Autodesk Fusion 360 part; units mm, degrees
(part 2 of 3)
  spline S15 degree 5 poles (-10.6114, -19.2717) (-10.6024, -19.2665) (-10.5842, -19.256) (-10.557, -19.2403) (-10.5209, -19.2193) (-10.476, -19.1928) (-10.4312, -19.1661) (-10.3866, -19.1393) (-10.3422, -19.1123) (-10.298, -19.0851) (-10.254, -19.0578) (-10.2102, -19.0302) (-10.1666, -19.0026) (-10.1231, -18.9747) (-10.0799, -18.9466) (-10.0369, -18.9184) (-9.9941, -18.8901) (-9.9515, -18.8615) (-9.9091, -18.8328) (-9.8669, -18.8038) (-9.8249, -18.7748) (-9.7832, -18.7455) (-9.7416, -18.7161) (-9.7003, -18.6865) (-9.6592, -18.6567) (-9.6183, -18.6267) (-9.5776, -18.5966) (-9.5372, -18.5662) (-9.497, -18.5357) (-9.457, -18.5051) (-9.4173, -18.4742) (-9.3778, -18.4432) (-9.3385, -18.412) (-9.2995, -18.3806) (-9.2607, -18.349) (-9.2222, -18.3172) (-9.1839, -18.2853) (-9.1459, -18.2531) (-9.1082, -18.2208) (-9.0707, -18.1883) (-9.0335, -18.1556) (-8.9965, -18.1227) (-8.9598, -18.0896) (-8.9234, -18.0564) (-8.8873, -18.0229) (-8.8515, -17.9892) (-8.816, -17.9554) (-8.7808, -17.9213) (-8.7458, -17.8871) (-8.7112, -17.8526) (-8.6769, -17.8179) (-8.643, -17.7831) (-8.6093, -17.748) (-8.576, -17.7127) (-8.5431, -17.6772) (-8.5105, -17.6415) (-8.4782, -17.6055) (-8.4464, -17.5693) (-8.415, -17.5329) (-8.384, -17.4962) (-8.3534, -17.4593) (-8.3232, -17.4221) (-8.2934, -17.3847) (-8.264, -17.3471) (-8.2352, -17.3092) (-8.2069, -17.2709) (-8.1792, -17.2323) (-8.1523, -17.1934) (-8.1261, -17.154) (-8.1007, -17.1142) (-8.0762, -17.074) (-8.0573, -17.0414) (-8.0434, -17.0168) (-8.0344, -17.0003) (-8.0299, -16.992) knots -1 -1 -1 -1 -1 -1 -0.98571429 -0.97142857 -0.95714286 -0.94285714 -0.92857143 -0.91428571 -0.9 -0.88571429 -0.87142857 -0.85714286 -0.84285714 -0.82857143 -0.81428571 -0.8 -0.78571429 -0.77142857 -0.75714286 -0.74285714 -0.72857143 -0.71428571 -0.7 -0.68571429 -0.67142857 -0.65714286 -0.64285714 -0.62857143 -0.61428571 -0.6 -0.58571429 -0.57142857 -0.55714286 -0.54285714 -0.52857143 -0.51428571 -0.5 -0.48571429 -0.47142857 -0.45714286 -0.44285714 -0.42857143 -0.41428571 -0.4 -0.38571429 -0.37142857 -0.35714286 -0.34285714 -0.32857143 -0.31428571 -0.3 -0.28571429 -0.27142857 -0.25714286 -0.24285714 -0.22857143 -0.21428571 -0.2 -0.18571429 -0.17142857 -0.15714286 -0.14285714 -0.12857143 -0.11428571 -0.1 -0.08571429 -0.07142857 -0.05714286 -0.04285714 -0.02857143 -0.01428571 0 0 0 0 0 0
  line L31 (-8.0299, -16.992) -> (-7.6878, -16.268)
  arc A23 (-7.0347, -16.0238) -> (-7.6878, -16.268) centre (-7.2357, -16.4816) ccw
  arc A24 (-7.0347, -16.0238) -> (-5.868, -16.4869) centre (0, 0) ccw
  arc A25 (-5.5602, -17.1124) -> (-5.868, -16.4869) centre (-6.0357, -16.9579) ccw
  line L32 (-5.5602, -17.1124) -> (-5.8076, -17.874)
  spline S16 degree 5 poles (-5.8076, -17.874) (-5.81, -17.8831) (-5.8148, -17.9013) (-5.8216, -17.9287) (-5.8301, -17.9654) (-5.8399, -18.0115) (-5.8487, -18.0579) (-5.8566, -18.1045) (-5.8637, -18.1513) (-5.8701, -18.1983) (-5.8757, -18.2456) (-5.8807, -18.293) (-5.8852, -18.3405) (-5.8891, -18.3882) (-5.8926, -18.4359) (-5.8957, -18.4838) (-5.8982, -18.5317) (-5.9003, -18.5798) (-5.902, -18.628) (-5.9032, -18.6762) (-5.904, -18.7246) (-5.9043, -18.773) (-5.9043, -18.8216) (-5.9039, -18.8702) (-5.903, -18.9188) (-5.9019, -18.9676) (-5.9003, -19.0164) (-5.8984, -19.0653) (-5.8961, -19.1142) (-5.8935, -19.1632) (-5.8905, -19.2123) (-5.8871, -19.2614) (-5.8835, -19.3106) (-5.8794, -19.3598) (-5.8751, -19.4091) (-5.8704, -19.4584) (-5.8654, -19.5078) (-5.8601, -19.5572) (-5.8545, -19.6066) (-5.8486, -19.6561) (-5.8423, -19.7057) (-5.8357, -19.7552) (-5.8289, -19.8048) (-5.8217, -19.8545) (-5.8142, -19.9042) (-5.8065, -19.9539) (-5.7984, -20.0036) (-5.7901, -20.0534) (-5.7814, -20.1032) (-5.7725, -20.153) (-5.7633, -20.2029) (-5.7538, -20.2527) (-5.744, -20.3026) (-5.734, -20.3525) (-5.7236, -20.4025) (-5.713, -20.4524) (-5.7021, -20.5024) (-5.691, -20.5524) (-5.6796, -20.6024) (-5.6679, -20.6524) (-5.6559, -20.7024) (-5.6437, -20.7525) (-5.6312, -20.8026) (-5.6184, -20.8526) (-5.6054, -20.9027) (-5.5921, -20.9528) (-5.5786, -21.0029) (-5.5648, -21.053) (-5.5507, -21.1031) (-5.5364, -21.1532) (-5.5219, -21.2033) (-5.51, -21.2434) (-5.501, -21.2734) (-5.4949, -21.2935) (-5.4919, -21.3035) knots 0 0 0 0 0 0 0.01428571 0.02857143 0.04285714 0.05714286 0.07142857 0.08571429 0.1 0.11428571 0.12857143 0.14285714 0.15714286 0.17142857 0.18571429 0.2 0.21428571 0.22857143 0.24285714 0.25714286 0.27142857 0.28571429 0.3 0.31428571 0.32857143 0.34285714 0.35714286 0.37142857 0.38571429 0.4 0.41428571 0.42857143 0.44285714 0.45714286 0.47142857 0.48571429 0.5 0.51428571 0.52857143 0.54285714 0.55714286 0.57142857 0.58571429 0.6 0.61428571 0.62857143 0.64285714 0.65714286 0.67142857 0.68571429 0.7 0.71428571 0.72857143 0.74285714 0.75714286 0.77142857 0.78571429 0.8 0.81428571 0.82857143 0.84285714 0.85714286 0.87142857 0.88571429 0.9 0.91428571 0.92857143 0.94285714 0.95714286 0.97142857 0.98571429 1 1 1 1 1 1
  line L33 (-5.4919, -21.3035) -> (-4.8168, -21.4662)
  line L34 (-4.8168, -21.4662) -> (-4.1368, -21.6076)
  spline S17 degree 5 poles (-4.1368, -21.6076) (-4.1298, -21.5998) (-4.1157, -21.5843) (-4.0948, -21.5609) (-4.0669, -21.5297) (-4.0323, -21.4907) (-3.998, -21.4515) (-3.9639, -21.4122) (-3.93, -21.3728) (-3.8964, -21.3333) (-3.863, -21.2937) (-3.8298, -21.254) (-3.7969, -21.2141) (-3.7642, -21.1742) (-3.7317, -21.1342) (-3.6996, -21.0941) (-3.6676, -21.0539) (-3.6359, -21.0135) (-3.6045, -20.9731) (-3.5733, -20.9326) (-3.5423, -20.8919) (-3.5117, -20.8512) (-3.4812, -20.8104) (-3.4511, -20.7694) (-3.4212, -20.7284) (-3.3916, -20.6873) (-3.3622, -20.646) (-3.3331, -20.6047) (-3.3043, -20.5633) (-3.2758, -20.5217) (-3.2475, -20.4801) (-3.2195, -20.4384) (-3.1918, -20.3966) (-3.1644, -20.3546) (-3.1373, -20.3126) (-3.1105, -20.2705) (-3.084, -20.2283) (-3.0578, -20.186) (-3.0318, -20.1436) (-3.0062, -20.1011) (-2.9809, -20.0585) (-2.956, -20.0158) (-2.9313, -19.973) (-2.907, -19.9301) (-2.883, -19.8871) (-2.8593, -19.844) (-2.836, -19.8009) (-2.813, -19.7576) (-2.7904, -19.7142) (-2.7681, -19.6708) (-2.7462, -19.6272) (-2.7247, -19.5835) (-2.7035, -19.5398) (-2.6828, -19.4959) (-2.6624, -19.452) (-2.6424, -19.4079) (-2.6229, -19.3638) (-2.6038, -19.3195) (-2.5852, -19.2751) (-2.567, -19.2307) (-2.5493, -19.1861) (-2.5321, -19.1414) (-2.5153, -19.0967) (-2.499, -19.0518) (-2.4833, -19.0068) (-2.4682, -18.9617) (-2.4538, -18.9164) (-2.4402, -18.8711) (-2.4275, -18.8255) (-2.4157, -18.7798) (-2.4048, -18.734) (-2.3968, -18.6972) (-2.3913, -18.6695) (-2.3878, -18.651) (-2.3861, -18.6418) knots -1 -1 -1 -1 -1 -1 -0.98571429 -0.97142857 -0.95714286 -0.94285714 -0.92857143 -0.91428571 -0.9 -0.88571429 -0.87142857 -0.85714286 -0.84285714 -0.82857143 -0.81428571 -0.8 -0.78571429 -0.77142857 -0.75714286 -0.74285714 -0.72857143 -0.71428571 -0.7 -0.68571429 -0.67142857 -0.65714286 -0.64285714 -0.62857143 -0.61428571 -0.6 -0.58571429 -0.57142857 -0.55714286 -0.54285714 -0.52857143 -0.51428571 -0.5 -0.48571429 -0.47142857 -0.45714286 -0.44285714 -0.42857143 -0.41428571 -0.4 -0.38571429 -0.37142857 -0.35714286 -0.34285714 -0.32857143 -0.31428571 -0.3 -0.28571429 -0.27142857 -0.25714286 -0.24285714 -0.22857143 -0.21428571 -0.2 -0.18571429 -0.17142857 -0.15714286 -0.14285714 -0.12857143 -0.11428571 -0.1 -0.08571429 -0.07142857 -0.05714286 -0.04285714 -0.02857143 -0.01428571 0 0 0 0 0 0
  line L35 (-2.3861, -18.6418) -> (-2.2844, -17.8474)
  arc A26 (-1.7388, -17.4134) -> (-2.2844, -17.8474) centre (-1.7885, -17.9109) ccw
  arc A27 (-1.7388, -17.4134) -> (-0.4861, -17.4932) centre (0, 0) ccw
  arc A28 (0, -17.9931) -> (-0.4861, -17.4932) centre (-0.5, -17.9931) ccw
  line L36 (0, -17.9931) -> (0, -18.7939)
  spline S18 degree 5 poles (0, -18.7939) (0.0005, -18.8032) (0.0016, -18.822) (0.0036, -18.8502) (0.0068, -18.8877) (0.0118, -18.9346) (0.0178, -18.9814) (0.0246, -19.0282) (0.0323, -19.0749) (0.0408, -19.1216) (0.0501, -19.1683) (0.06, -19.2149) (0.0704, -19.2615) (0.0814, -19.308) (0.0928, -19.3545) (0.1047, -19.401) (0.1171, -19.4474) (0.1299, -19.4937) (0.1432, -19.5401) (0.157, -19.5863) (0.1712, -19.6326) (0.1858, -19.6788) (0.2009, -19.7249) (0.2163, -19.771) (0.2321, -19.817) (0.2483, -19.863) (0.2649, -19.909) (0.2818, -19.9549) (0.2991, -20.0007) (0.3167, -20.0465) (0.3347, -20.0922) (0.3531, -20.1379) (0.3718, -20.1835) (0.3908, -20.2291) (0.4102, -20.2746) (0.4299, -20.3201) (0.4499, -20.3655) (0.4702, -20.4109) (0.4908, -20.4561) (0.5118, -20.5014) (0.533, -20.5466) (0.5546, -20.5917) (0.5764, -20.6367) (0.5986, -20.6817) (0.6211, -20.7267) (0.6438, -20.7716) (0.6668, -20.8164) (0.6902, -20.8611) (0.7138, -20.9058) (0.7376, -20.9504) (0.7618, -20.995) (0.7863, -21.0395) (0.811, -21.0839) (0.836, -21.1283) (0.8612, -21.1726) (0.8867, -21.2168) (0.9125, -21.261) (0.9386, -21.3051) (0.9649, -21.3491) (0.9915, -21.3931) (1.0183, -21.437) (1.0454, -21.4808) (1.0728, -21.5245) (1.1004, -21.5682) (1.1282, -21.6118) (1.1563, -21.6553) (1.1847, -21.6988) (1.2133, -21.7422) (1.2421, -21.7855) (1.2712, -21.8287) (1.3006, -21.8719) (1.3242, -21.9063) (1.3421, -21.9321) (1.354, -21.9493) (1.36, -21.9579) knots 0 0 0 0 0 0 0.01428571 0.02857143 0.04285714 0.05714286 0.07142857 0.08571429 0.1 0.11428571 0.12857143 0.14285714 0.15714286 0.17142857 0.18571429 0.2 0.21428571 0.22857143 0.24285714 0.25714286 0.27142857 0.28571429 0.3 0.31428571 0.32857143 0.34285714 0.35714286 0.37142857 0.38571429 0.4 0.41428571 0.42857143 0.44285714 0.45714286 0.47142857 0.48571429 0.5 0.51428571 0.52857143 0.54285714 0.55714286 0.57142857 0.58571429 0.6 0.61428571 0.62857143 0.64285714 0.65714286 0.67142857 0.68571429 0.7 0.71428571 0.72857143 0.74285714 0.75714286 0.77142857 0.78571429 0.8 0.81428571 0.82857143 0.84285714 0.85714286 0.87142857 0.88571429 0.9 0.91428571 0.92857143 0.94285714 0.95714286 0.97142857 0.98571429 1 1 1 1 1 1
  line L37 (1.36, -21.9579) -> (2.0524, -21.9041)
  line L38 (2.0524, -21.9041) -> (2.7428, -21.8284)
  spline S19 degree 5 poles (2.7428, -21.8284) (2.747, -21.8188) (2.7556, -21.7997) (2.7683, -21.771) (2.7852, -21.7327) (2.806, -21.6849) (2.8265, -21.637) (2.8468, -21.5891) (2.8669, -21.5412) (2.8867, -21.4932) (2.9062, -21.4452) (2.9255, -21.3972) (2.9445, -21.3491) (2.9632, -21.3011) (2.9817, -21.253) (2.9999, -21.2049) (3.0179, -21.1568) (3.0356, -21.1086) (3.053, -21.0604) (3.0701, -21.0123) (3.087, -20.964) (3.1036, -20.9158) (3.1199, -20.8676) (3.1359, -20.8193) (3.1517, -20.7711) (3.1672, -20.7228) (3.1823, -20.6745) (3.1972, -20.6262) (3.2118, -20.5779) (3.2261, -20.5296) (3.2401, -20.4813) (3.2539, -20.4329) (3.2673, -20.3846) (3.2804, -20.3363) (3.2932, -20.2879) (3.3057, -20.2396) (3.3179, -20.1913) (3.3297, -20.1429) (3.3413, -20.0946) (3.3525, -20.0462) (3.3634, -19.9979) (3.3739, -19.9496) (3.3842, -19.9013) (3.3941, -19.853) (3.4036, -19.8047) (3.4128, -19.7564) (3.4216, -19.7081) (3.4301, -19.6599) (3.4382, -19.6116) (3.446, -19.5634) (3.4533, -19.5152) (3.4603, -19.467) (3.4669, -19.4189) (3.4731, -19.3707) (3.4789, -19.3226) (3.4843, -19.2746) (3.4892, -19.2265) (3.4937, -19.1786) (3.4977, -19.1306) (3.5012, -19.0827) (3.5043, -19.0349) (3.5069, -18.987) (3.509, -18.9393) (3.5106, -18.8916) (3.5117, -18.8439) (3.5121, -18.7963) (3.5118, -18.7489) (3.5107, -18.7015) (3.5087, -18.6543) (3.5058, -18.6072) (3.502, -18.5602) (3.4982, -18.5227) (3.4949, -18.4947) (3.4926, -18.476) (3.4913, -18.4667) knots -1 -1 -1 -1 -1 -1 -0.98571429 -0.97142857 -0.95714286 -0.94285714 -0.92857143 -0.91428571 -0.9 -0.88571429 -0.87142857 -0.85714286 -0.84285714 -0.82857143 -0.81428571 -0.8 -0.78571429 -0.77142857 -0.75714286 -0.74285714 -0.72857143 -0.71428571 -0.7 -0.68571429 -0.67142857 -0.65714286 -0.64285714 -0.62857143 -0.61428571 -0.6 -0.58571429 -0.57142857 -0.55714286 -0.54285714 -0.52857143 -0.51428571 -0.5 -0.48571429 -0.47142857 -0.45714286 -0.44285714 -0.42857143 -0.41428571 -0.4 -0.38571429 -0.37142857 -0.35714286 -0.34285714 -0.32857143 -0.31428571 -0.3 -0.28571429 -0.27142857 -0.25714286 -0.24285714 -0.22857143 -0.21428571 -0.2 -0.18571429 -0.17142857 -0.15714286 -0.14285714 -0.12857143 -0.11428571 -0.1 -0.08571429 -0.07142857 -0.05714286 -0.04285714 -0.02857143 -0.01428571 0 0 0 0 0 0
  line L39 (3.4913, -18.4667) -> (3.3426, -17.6799)
  arc A29 (3.7274, -17.0984) -> (3.3426, -17.6799) centre (3.8339, -17.587) ccw
  arc A30 (3.7274, -17.0984) -> (4.9434, -16.7873) centre (0, 0) ccw
  arc A31 (5.5602, -17.1124) -> (4.9434, -16.7873) centre (5.0846, -17.2669) ccw
  line L40 (5.5602, -17.1124) -> (5.8076, -17.874)
  spline S20 degree 5 poles (5.8076, -17.874) (5.811, -17.8828) (5.8179, -17.9003) (5.8285, -17.9265) (5.8431, -17.9612) (5.8623, -18.0042) (5.8825, -18.0469) (5.9034, -18.0893) (5.9252, -18.1313) (5.9477, -18.1731) (5.9709, -18.2146) (5.9947, -18.2559) (6.0191, -18.297) (6.0439, -18.3379) (6.0691, -18.3786) (6.0948, -18.4191) (6.1209, -18.4594) (6.1475, -18.4995) (6.1744, -18.5395) (6.2018, -18.5792) (6.2296, -18.6188) (6.2578, -18.6582) (6.2864, -18.6974) (6.3153, -18.7365) (6.3445, -18.7754) (6.3742, -18.8141) (6.4041, -18.8527) (6.4344, -18.8911) (6.465, -18.9294) (6.4959, -18.9675) (6.5272, -19.0054) (6.5588, -19.0432) (6.5907, -19.0808) (6.6228, -19.1183) (6.6553, -19.1556) (6.6881, -19.1927) (6.7211, -19.2297) (6.7545, -19.2666) (6.7881, -19.3033) (6.822, -19.3398) (6.8562, -19.3762) (6.8906, -19.4125) (6.9253, -19.4486) (6.9603, -19.4845) (6.9956, -19.5203) (7.0311, -19.556) (7.0668, -19.5915) (7.1028, -19.6268) (7.1391, -19.6621) (7.1756, -19.6971) (7.2123, -19.732) (7.2493, -19.7668) (7.2866, -19.8014) (7.324, -19.8359) (7.3618, -19.8702) (7.3997, -19.9044) (7.4379, -19.9384) (7.4763, -19.9723) (7.5149, -20.006) (7.5538, -20.0396) (7.5929, -20.0731) (7.6322, -20.1064) (7.6717, -20.1395) (7.7115, -20.1725) (7.7514, -20.2054) (7.7916, -20.2381) (7.832, -20.2707) (7.8726, -20.3031) (7.9134, -20.3354) (7.9545, -20.3675) (7.9957, -20.3995) (8.0288, -20.4249) (8.0538, -20.444) (8.0705, -20.4566) (8.0788, -20.463) knots 0 0 0 0 0 0 0.01428571 0.02857143 0.04285714 0.05714286 0.07142857 0.08571429 0.1 0.11428571 0.12857143 0.14285714 0.15714286 0.17142857 0.18571429 0.2 0.21428571 0.22857143 0.24285714 0.25714286 0.27142857 0.28571429 0.3 0.31428571 0.32857143 0.34285714 0.35714286 0.37142857 0.38571429 0.4 0.41428571 0.42857143 0.44285714 0.45714286 0.47142857 0.48571429 0.5 0.51428571 0.52857143 0.54285714 0.55714286 0.57142857 0.58571429 0.6 0.61428571 0.62857143 0.64285714 0.65714286 0.67142857 0.68571429 0.7 0.71428571 0.72857143 0.74285714 0.75714286 0.77142857 0.78571429 0.8 0.81428571 0.82857143 0.84285714 0.85714286 0.87142857 0.88571429 0.9 0.91428571 0.92857143 0.94285714 0.95714286 0.97142857 0.98571429 1 1 1 1 1 1
  line L41 (8.0788, -20.463) -> (8.7207, -20.1978)
  line L42 (8.7207, -20.1978) -> (9.3539, -19.9124)
  spline S21 degree 5 poles (9.3539, -19.9124) (9.355, -19.902) (9.3572, -19.8812) (9.3605, -19.85) (9.3647, -19.8084) (9.3697, -19.7565) (9.3744, -19.7046) (9.3789, -19.6527) (9.3832, -19.6009) (9.3872, -19.5492) (9.3909, -19.4975) (9.3944, -19.4459) (9.3976, -19.3943) (9.4006, -19.3428) (9.4033, -19.2914) (9.4058, -19.24) (9.408, -19.1887) (9.4099, -19.1374) (9.4116, -19.0862) (9.413, -19.0351) (9.4142, -18.9841) (9.415, -18.9331) (9.4156, -18.8822) (9.416, -18.8313) (9.416, -18.7805) (9.4158, -18.7299) (9.4154, -18.6792) (9.4146, -18.6287) (9.4136, -18.5783) (9.4122, -18.5279) (9.4106, -18.4776) (9.4087, -18.4274) (9.4065, -18.3773) (9.4041, -18.3273) (9.4013, -18.2773) (9.3983, -18.2275) (9.3949, -18.1778) (9.3913, -18.1281) (9.3873, -18.0786) (9.383, -18.0291) (9.3784, -17.9798) (9.3736, -17.9306) (9.3684, -17.8815) (9.3628, -17.8325) (9.357, -17.7836) (9.3508, -17.7348) (9.3443, -17.6862) (9.3375, -17.6377) (9.3303, -17.5893) (9.3227, -17.541) (9.3148, -17.4929) (9.3066, -17.4449) (9.298, -17.3971) (9.289, -17.3494) (9.2797, -17.3019) (9.2699, -17.2545) (9.2598, -17.2073) (9.2492, -17.1603) (9.2382, -17.1134) (9.2267, -17.0668) (9.2149, -17.0203) (9.2026, -16.9741) (9.1898, -16.928) (9.1766, -16.8821) (9.1629, -16.8365) (9.1486, -16.7911) (9.1336, -16.746) (9.1179, -16.7013) (9.1015, -16.657) (9.0842, -16.6131) (9.066, -16.5696) (9.0508, -16.5352) (9.0391, -16.5095) (9.031, -16.4925) (9.027, -16.484) knots -1 -1 -1 -1 -1 -1 -0.98571429 -0.97142857 -0.95714286 -0.94285714 -0.92857143 -0.91428571 -0.9 -0.88571429 -0.87142857 -0.85714286 -0.84285714 -0.82857143 -0.81428571 -0.8 -0.78571429 -0.77142857 -0.75714286 -0.74285714 -0.72857143 -0.71428571 -0.7 -0.68571429 -0.67142857 -0.65714286 -0.64285714 -0.62857143 -0.61428571 -0.6 -0.58571429 -0.57142857 -0.55714286 -0.54285714 -0.52857143 -0.51428571 -0.5 -0.48571429 -0.47142857 -0.45714286 -0.44285714 -0.42857143 -0.41428571 -0.4 -0.38571429 -0.37142857 -0.35714286 -0.34285714 -0.32857143 -0.31428571 -0.3 -0.28571429 -0.27142857 -0.25714286 -0.24285714 -0.22857143 -0.21428571 -0.2 -0.18571429 -0.17142857 -0.15714286 -0.14285714 -0.12857143 -0.11428571 -0.1 -0.08571429 -0.07142857 -0.05714286 -0.04285714 -0.02857143 -0.01428571 0 0 0 0 0 0
  line L43 (9.027, -16.484) -> (8.6423, -15.7816)
  arc A32 (8.8286, -15.1098) -> (8.6423, -15.7816) centre (9.0809, -15.5415) ccw
  arc A33 (8.8286, -15.1098) -> (9.889, -14.4381) centre (0, 0) ccw
  arc A34 (10.5761, -14.5567) -> (9.889, -14.4381) centre (10.1715, -14.8506) ccw
  line L44 (10.5761, -14.5567) -> (11.0467, -15.2045)
  spline S22 degree 5 poles (11.0467, -15.2045) (11.0527, -15.2118) (11.0646, -15.2264) (11.0828, -15.248) (11.1074, -15.2764) (11.139, -15.3114) (11.1713, -15.3458) (11.2044, -15.3796) (11.2381, -15.4129) (11.2724, -15.4457) (11.3073, -15.478) (11.3427, -15.5099) (11.3786, -15.5415) (11.4148, -15.5727) (11.4514, -15.6036) (11.4883, -15.6342) (11.5256, -15.6644) (11.5632, -15.6944) (11.6012, -15.7241) (11.6396, -15.7534) (11.6782, -15.7825) (11.7172, -15.8112) (11.7565, -15.8397) (11.7961, -15.8679) (11.8359, -15.8959) (11.8761, -15.9236) (11.9165, -15.951) (11.9571, -15.9782) (11.9981, -16.0051) (12.0393, -16.0318) (12.0807, -16.0582) (12.1224, -16.0844) (12.1644, -16.1103) (12.2066, -16.136) (12.249, -16.1614) (12.2916, -16.1866) (12.3345, -16.2116) (12.3776, -16.2364) (12.4209, -16.2609) (12.4644, -16.2852) (12.5082, -16.3092) (12.5522, -16.333) (12.5963, -16.3567) (12.6407, -16.38) (12.6853, -16.4032) (12.7301, -16.4261) (12.775, -16.4489) (12.8202, -16.4713) (12.8656, -16.4936) (12.9111, -16.5157) (12.9569, -16.5375) (13.0028, -16.5592) (13.0489, -16.5806) (13.0952, -16.6018) (13.1417, -16.6228) (13.1883, -16.6436) (13.2352, -16.6641) (13.2822, -16.6845) (13.3293, -16.7046) (13.3767, -16.7246) (13.4242, -16.7443) (13.4719, -16.7638) (13.5197, -16.7831) (13.5677, -16.8023) (13.6159, -16.8212) (13.6642, -16.8398) (13.7127, -16.8583) (13.7613, -16.8766) (13.8101, -16.8947) (13.859, -16.9126) (13.9081, -16.9302) (13.9475, -16.9442) (13.9772, -16.9546) (13.9969, -16.9615) (14.0068, -16.9649) knots 0 0 0 0 0 0 0.01428571 0.02857143 0.04285714 0.05714286 0.07142857 0.08571429 0.1 0.11428571 0.12857143 0.14285714 0.15714286 0.17142857 0.18571429 0.2 0.21428571 0.22857143 0.24285714 0.25714286 0.27142857 0.28571429 0.3 0.31428571 0.32857143 0.34285714 0.35714286 0.37142857 0.38571429 0.4 0.41428571 0.42857143 0.44285714 0.45714286 0.47142857 0.48571429 0.5 0.51428571 0.52857143 0.54285714 0.55714286 0.57142857 0.58571429 0.6 0.61428571 0.62857143 0.64285714 0.65714286 0.67142857 0.68571429 0.7 0.71428571 0.72857143 0.74285714 0.75714286 0.77142857 0.78571429 0.8 0.81428571 0.82857143 0.84285714 0.85714286 0.87142857 0.88571429 0.9 0.91428571 0.92857143 0.94285714 0.95714286 0.97142857 0.98571429 1 1 1 1 1 1
  line L45 (14.0068, -16.9649) -> (14.5353, -16.5144)
  line L46 (14.5353, -16.5144) -> (15.0493, -16.0474)
  spline S23 degree 5 poles (15.0493, -16.0474) (15.0472, -16.0371) (15.0429, -16.0166) (15.0363, -15.9859) (15.0275, -15.9451) (15.0162, -15.8941) (15.0046, -15.8433) (14.9929, -15.7926) (14.9809, -15.7421) (14.9688, -15.6916) (14.9564, -15.6413) (14.9437, -15.5911) (14.9309, -15.5411) (14.9178, -15.4912) (14.9045, -15.4414) (14.8909, -15.3918) (14.8772, -15.3423) (14.8632, -15.293) (14.8489, -15.2437) (14.8345, -15.1947) (14.8198, -15.1458) (14.8049, -15.097) (14.7897, -15.0484) (14.7743, -14.9999) (14.7587, -14.9516) (14.7428, -14.9035) (14.7267, -14.8555) (14.7104, -14.8077) (14.6938, -14.76) (14.677, -14.7125) (14.6599, -14.6652) (14.6426, -14.618) (14.6251, -14.571) (14.6072, -14.5242) (14.5892, -14.4776) (14.5709, -14.4312) (14.5523, -14.3849) (14.5335, -14.3388) (14.5144, -14.2929) (14.4951, -14.2472) (14.4755, -14.2017) (14.4556, -14.1564) (14.4355, -14.1113) (14.4151, -14.0664) (14.3945, -14.0217) (14.3735, -13.9773) (14.3523, -13.933) (14.3308, -13.889) (14.309, -13.8452) (14.2869, -13.8016) (14.2645, -13.7583) (14.2419, -13.7152) (14.2189, -13.6724) (14.1956, -13.6298) (14.1721, -13.5875) (14.1482, -13.5454) (14.1239, -13.5037) (14.0993, -13.4622) (14.0744, -13.4211) (14.0491, -13.3803) (14.0234, -13.3397) (13.9974, -13.2995) (13.9711, -13.2596) (13.9443, -13.2201) (13.9172, -13.1809) (13.8896, -13.1422) (13.8614, -13.104) (13.8327, -13.0663) (13.8033, -13.0293) (13.7733, -12.9928) (13.7426, -12.9571) (13.7175, -12.929) (13.6984, -12.9083) (13.6855, -12.8946) (13.679, -12.8877) knots -1 -1 -1 -1 -1 -1 -0.98571429 -0.97142857 -0.95714286 -0.94285714 -0.92857143 -0.91428571 -0.9 -0.88571429 -0.87142857 -0.85714286 -0.84285714 -0.82857143 -0.81428571 -0.8 -0.78571429 -0.77142857 -0.75714286 -0.74285714 -0.72857143 -0.71428571 -0.7 -0.68571429 -0.67142857 -0.65714286 -0.64285714 -0.62857143 -0.61428571 -0.6 -0.58571429 -0.57142857 -0.55714286 -0.54285714 -0.52857143 -0.51428571 -0.5 -0.48571429 -0.47142857 -0.45714286 -0.44285714 -0.42857143 -0.41428571 -0.4 -0.38571429 -0.37142857 -0.35714286 -0.34285714 -0.32857143 -0.31428571 -0.3 -0.28571429 -0.27142857 -0.25714286 -0.24285714 -0.22857143 -0.21428571 -0.2 -0.18571429 -0.17142857 -0.15714286 -0.14285714 -0.12857143 -0.11428571 -0.1 -0.08571429 -0.07142857 -0.05714286 -0.04285714 -0.02857143 -0.01428571 0 0 0 0 0 0
  line L47 (13.679, -12.8877) -> (13.0961, -12.3386)
  arc A35 (13.0657, -11.642) -> (13.0961, -12.3386) centre (13.439, -11.9747) ccw
  arc A36 (13.0657, -11.642) -> (13.8666, -10.6755) centre (0, 0) ccw
  arc A37 (14.5567, -10.5761) -> (13.8666, -10.6755) centre (14.2628, -10.9806) ccw
  line L48 (14.5567, -10.5761) -> (15.2045, -11.0467)
  spline S24 degree 5 poles (15.2045, -11.0467) (15.2124, -11.0519) (15.2283, -11.062) (15.2522, -11.0769) (15.2845, -11.0964) (15.3253, -11.1199) (15.3667, -11.1426) (15.4086, -11.1646) (15.4509, -11.1858) (15.4937, -11.2064) (15.5369, -11.2263) (15.5804, -11.2457) (15.6242, -11.2647) (15.6683, -11.2831) (15.7127, -11.3012) (15.7573, -11.3189) (15.8021, -11.3362) (15.8471, -11.353) (15.8924, -11.3695) (15.938, -11.3856) (15.9837, -11.4012) (16.0297, -11.4165) (16.0758, -11.4315) (16.1222, -11.4461) (16.1687, -11.4604) (16.2155, -11.4743) (16.2624, -11.4879) (16.3094, -11.5012) (16.3567, -11.5141) (16.4041, -11.5268) (16.4517, -11.5391) (16.4995, -11.5511) (16.5474, -11.5628) (16.5954, -11.5742) (16.6436, -11.5853) (16.692, -11.5961) (16.7405, -11.6066) (16.7891, -11.6168) (16.8379, -11.6267) (16.8868, -11.6364) (16.9358, -11.6457) (16.985, -11.6548) (17.0343, -11.6636) (17.0837, -11.6721) (17.1333, -11.6804) (17.183, -11.6884) (17.2328, -11.6961) (17.2827, -11.7035) (17.3327, -11.7107) (17.3828, -11.7176) (17.4331, -11.7242) (17.4835, -11.7306) (17.5339, -11.7367) (17.5845, -11.7426) (17.6352, -11.7482) (17.686, -11.7536) (17.7369, -11.7586) (17.7879, -11.7635) (17.839, -11.7681) (17.8902, -11.7724) (17.9414, -11.7765) (17.9928, -11.7803) (18.0443, -11.7839) (18.0958, -11.7872) (18.1475, -11.7903) (18.1992, -11.7932) (18.251, -11.7958) (18.3029, -11.7981) (18.3549, -11.8003) (18.407, -11.8021) (18.4592, -11.8038) (18.5009, -11.8049) (18.5323, -11.8056) (18.5533, -11.8061) (18.5637, -11.8063) knots 0 0 0 0 0 0 0.01428571 0.02857143 0.04285714 0.05714286 0.07142857 0.08571429 0.1 0.11428571 0.12857143 0.14285714 0.15714286 0.17142857 0.18571429 0.2 0.21428571 0.22857143 0.24285714 0.25714286 0.27142857 0.28571429 0.3 0.31428571 0.32857143 0.34285714 0.35714286 0.37142857 0.38571429 0.4 0.41428571 0.42857143 0.44285714 0.45714286 0.47142857 0.48571429 0.5 0.51428571 0.52857143 0.54285714 0.55714286 0.57142857 0.58571429 0.6 0.61428571 0.62857143 0.64285714 0.65714286 0.67142857 0.68571429 0.7 0.71428571 0.72857143 0.74285714 0.75714286 0.77142857 0.78571429 0.8 0.81428571 0.82857143 0.84285714 0.85714286 0.87142857 0.88571429 0.9 0.91428571 0.92857143 0.94285714 0.95714286 0.97142857 0.98571429 1 1 1 1 1 1
  line L49 (18.5637, -11.8063) -> (18.9271, -11.2144)
  line L50 (18.9271, -11.2144) -> (19.2717, -10.6114)
  spline S25 degree 5 poles (19.2717, -10.6114) (19.2665, -10.6024) (19.256, -10.5842) (19.2403, -10.557) (19.2193, -10.5209) (19.1928, -10.476) (19.1661, -10.4312) (19.1393, -10.3866) (19.1123, -10.3422) (19.0851, -10.298) (19.0578, -10.254) (19.0302, -10.2102) (19.0026, -10.1666) (18.9747, -10.1231) (18.9466, -10.0799) (18.9184, -10.0369) (18.8901, -9.9941) (18.8615, -9.9515) (18.8328, -9.9091) (18.8038, -9.8669) (18.7748, -9.8249) (18.7455, -9.7832) (18.7161, -9.7416) (18.6865, -9.7003) (18.6567, -9.6592) (18.6267, -9.6183) (18.5966, -9.5776) (18.5662, -9.5372) (18.5357, -9.497) (18.5051, -9.457) (18.4742, -9.4173) (18.4432, -9.3778) (18.412, -9.3385) (18.3806, -9.2995) (18.349, -9.2607) (18.3172, -9.2222) (18.2853, -9.1839) (18.2531, -9.1459) (18.2208, -9.1082) (18.1883, -9.0707) (18.1556, -9.0335) (18.1227, -8.9965) (18.0896, -8.9598) (18.0564, -8.9234) (18.0229, -8.8873) (17.9892, -8.8515) (17.9554, -8.816) (17.9213, -8.7808) (17.8871, -8.7458) (17.8526, -8.7112) (17.8179, -8.6769) (17.7831, -8.643) (17.748, -8.6093) (17.7127, -8.576) (17.6772, -8.5431) (17.6415, -8.5105) (17.6055, -8.4782) (17.5693, -8.4464) (17.5329, -8.415) (17.4962, -8.384) (17.4593, -8.3534) (17.4221, -8.3232) (17.3847, -8.2934) (17.3471, -8.264) (17.3092, -8.2352) (17.2709, -8.2069) (17.2323, -8.1792) (17.1934, -8.1523) (17.154, -8.1261) (17.1142, -8.1007) (17.074, -8.0762) (17.0414, -8.0573) (17.0168, -8.0434) (17.0003, -8.0344) (16.992, -8.0299) knots -1 -1 -1 -1 -1 -1 -0.98571429 -0.97142857 -0.95714286 -0.94285714 -0.92857143 -0.91428571 -0.9 -0.88571429 -0.87142857 -0.85714286 -0.84285714 -0.82857143 -0.81428571 -0.8 -0.78571429 -0.77142857 -0.75714286 -0.74285714 -0.72857143 -0.71428571 -0.7 -0.68571429 -0.67142857 -0.65714286 -0.64285714 -0.62857143 -0.61428571 -0.6 -0.58571429 -0.57142857 -0.55714286 -0.54285714 -0.52857143 -0.51428571 -0.5 -0.48571429 -0.47142857 -0.45714286 -0.44285714 -0.42857143 -0.41428571 -0.4 -0.38571429 -0.37142857 -0.35714286 -0.34285714 -0.32857143 -0.31428571 -0.3 -0.28571429 -0.27142857 -0.25714286 -0.24285714 -0.22857143 -0.21428571 -0.2 -0.18571429 -0.17142857 -0.15714286 -0.14285714 -0.12857143 -0.11428571 -0.1 -0.08571429 -0.07142857 -0.05714286 -0.04285714 -0.02857143 -0.01428571 0 0 0 0 0 0
  line L51 (16.992, -8.0299) -> (16.268, -7.6878)
  arc A38 (16.0238, -7.0347) -> (16.268, -7.6878) centre (16.4816, -7.2357) ccw
  arc A39 (16.0238, -7.0347) -> (16.4869, -5.868) centre (0, 0) ccw
  arc A40 (17.1124, -5.5602) -> (16.4869, -5.868) centre (16.9579, -6.0357) ccw
  line L52 (17.1124, -5.5602) -> (17.874, -5.8076)
  spline S26 degree 5 poles (17.874, -5.8076) (17.8831, -5.81) (17.9013, -5.8148) (17.9287, -5.8216) (17.9654, -5.8301) (18.0115, -5.8399) (18.0579, -5.8487) (18.1045, -5.8566) (18.1513, -5.8637) (18.1983, -5.8701) (18.2456, -5.8757) (18.293, -5.8807) (18.3405, -5.8852) (18.3882, -5.8891) (18.4359, -5.8926) (18.4838, -5.8957) (18.5317, -5.8982) (18.5798, -5.9003) (18.628, -5.902) (18.6762, -5.9032) (18.7246, -5.904) (18.773, -5.9043) (18.8216, -5.9043) (18.8702, -5.9039) (18.9188, -5.903) (18.9676, -5.9019) (19.0164, -5.9003) (19.0653, -5.8984) (19.1142, -5.8961) (19.1632, -5.8935) (19.2123, -5.8905) (19.2614, -5.8871) (19.3106, -5.8835) (19.3598, -5.8794) (19.4091, -5.8751) (19.4584, -5.8704) (19.5078, -5.8654) (19.5572, -5.8601) (19.6066, -5.8545) (19.6561, -5.8486) (19.7057, -5.8423) (19.7552, -5.8357) (19.8048, -5.8289) (19.8545, -5.8217) (19.9042, -5.8142) (19.9539, -5.8065) (20.0036, -5.7984) (20.0534, -5.7901) (20.1032, -5.7814) (20.153, -5.7725) (20.2029, -5.7633) (20.2527, -5.7538) (20.3026, -5.744) (20.3525, -5.734) (20.4025, -5.7236) (20.4524, -5.713) (20.5024, -5.7021) (20.5524, -5.691) (20.6024, -5.6796) (20.6524, -5.6679) (20.7024, -5.6559) (20.7525, -5.6437) (20.8026, -5.6312) (20.8526, -5.6184) (20.9027, -5.6054) (20.9528, -5.5921) (21.0029, -5.5786) (21.053, -5.5648) (21.1031, -5.5507) (21.1532, -5.5364) (21.2033, -5.5219) (21.2434, -5.51) (21.2734, -5.501) (21.2935, -5.4949) (21.3035, -5.4919) knots 0 0 0 0 0 0 0.01428571 0.02857143 0.04285714 0.05714286 0.07142857 0.08571429 0.1 0.11428571 0.12857143 0.14285714 0.15714286 0.17142857 0.18571429 0.2 0.21428571 0.22857143 0.24285714 0.25714286 0.27142857 0.28571429 0.3 0.31428571 0.32857143 0.34285714 0.35714286 0.37142857 0.38571429 0.4 0.41428571 0.42857143 0.44285714 0.45714286 0.47142857 0.48571429 0.5 0.51428571 0.52857143 0.54285714 0.55714286 0.57142857 0.58571429 0.6 0.61428571 0.62857143 0.64285714 0.65714286 0.67142857 0.68571429 0.7 0.71428571 0.72857143 0.74285714 0.75714286 0.77142857 0.78571429 0.8 0.81428571 0.82857143 0.84285714 0.85714286 0.87142857 0.88571429 0.9 0.91428571 0.92857143 0.94285714 0.95714286 0.97142857 0.98571429 1 1 1 1 1 1
  line L53 (21.3035, -5.4919) -> (21.4662, -4.8168)
  line L54 (21.4662, -4.8168) -> (21.6076, -4.1368)
  spline S27 degree 5 poles (21.6076, -4.1368) (21.5998, -4.1298) (21.5843, -4.1157) (21.5609, -4.0948) (21.5297, -4.0669) (21.4907, -4.0323) (21.4515, -3.998) (21.4122, -3.9639) (21.3728, -3.93) (21.3333, -3.8964) (21.2937, -3.863) (21.254, -3.8298) (21.2141, -3.7969) (21.1742, -3.7642) (21.1342, -3.7317) (21.0941, -3.6996) (21.0539, -3.6676) (21.0135, -3.6359) (20.9731, -3.6045) (20.9326, -3.5733) (20.8919, -3.5423) (20.8512, -3.5117) (20.8104, -3.4812) (20.7694, -3.4511) (20.7284, -3.4212) (20.6873, -3.3916) (20.646, -3.3622) (20.6047, -3.3331) (20.5633, -3.3043) (20.5217, -3.2758) (20.4801, -3.2475) (20.4384, -3.2195) (20.3966, -3.1918) (20.3546, -3.1644) (20.3126, -3.1373) (20.2705, -3.1105) (20.2283, -3.084) (20.186, -3.0578) (20.1436, -3.0318) (20.1011, -3.0062) (20.0585, -2.9809) (20.0158, -2.956) (19.973, -2.9313) (19.9301, -2.907) (19.8871, -2.883) (19.844, -2.8593) (19.8009, -2.836) (19.7576, -2.813) (19.7142, -2.7904) (19.6708, -2.7681) (19.6272, -2.7462) (19.5835, -2.7247) (19.5398, -2.7035) (19.4959, -2.6828) (19.452, -2.6624) (19.4079, -2.6424) (19.3638, -2.6229) (19.3195, -2.6038) (19.2751, -2.5852) (19.2307, -2.567) (19.1861, -2.5493) (19.1414, -2.5321) (19.0967, -2.5153) (19.0518, -2.499) (19.0068, -2.4833) (18.9617, -2.4682) (18.9164, -2.4538) (18.8711, -2.4402) (18.8255, -2.4275) (18.7798, -2.4157) (18.734, -2.4048) (18.6972, -2.3968) (18.6695, -2.3913) (18.651, -2.3878) (18.6418, -2.3861) knots -1 -1 -1 -1 -1 -1 -0.98571429 -0.97142857 -0.95714286 -0.94285714 -0.92857143 -0.91428571 -0.9 -0.88571429 -0.87142857 -0.85714286 -0.84285714 -0.82857143 -0.81428571 -0.8 -0.78571429 -0.77142857 -0.75714286 -0.74285714 -0.72857143 -0.71428571 -0.7 -0.68571429 -0.67142857 -0.65714286 -0.64285714 -0.62857143 -0.61428571 -0.6 -0.58571429 -0.57142857 -0.55714286 -0.54285714 -0.52857143 -0.51428571 -0.5 -0.48571429 -0.47142857 -0.45714286 -0.44285714 -0.42857143 -0.41428571 -0.4 -0.38571429 -0.37142857 -0.35714286 -0.34285714 -0.32857143 -0.31428571 -0.3 -0.28571429 -0.27142857 -0.25714286 -0.24285714 -0.22857143 -0.21428571 -0.2 -0.18571429 -0.17142857 -0.15714286 -0.14285714 -0.12857143 -0.11428571 -0.1 -0.08571429 -0.07142857 -0.05714286 -0.04285714 -0.02857143 -0.01428571 0 0 0 0 0 0
  line L55 (18.6418, -2.3861) -> (17.8474, -2.2844)
  arc A41 (17.4134, -1.7388) -> (17.8474, -2.2844) centre (17.9109, -1.7885) ccw
  arc A42 (17.4134, -1.7388) -> (17.4932, -0.4861) centre (0, 0) ccw
  arc A43 (17.9931, 0) -> (17.4932, -0.4861) centre (17.9931, -0.5) ccw
  line L56 (17.9931, 0) -> (18.7939, 0)
  spline S28 degree 5 poles (18.7939, 0) (18.8032, 0.0005) (18.822, 0.0016) (18.8502, 0.0036) (18.8877, 0.0068) (18.9346, 0.0118) (18.9814, 0.0178) (19.0282, 0.0246) (19.0749, 0.0323) (19.1216, 0.0408) (19.1683, 0.0501) (19.2149, 0.06) (19.2615, 0.0704) (19.308, 0.0814) (19.3545, 0.0928) (19.401, 0.1047) (19.4474, 0.1171) (19.4937, 0.1299) (19.5401, 0.1432) (19.5863, 0.157) (19.6326, 0.1712) (19.6788, 0.1858) (19.7249, 0.2009) (19.771, 0.2163) (19.817, 0.2321) (19.863, 0.2483) (19.909, 0.2649) (19.9549, 0.2818) (20.0007, 0.2991) (20.0465, 0.3167) (20.0922, 0.3347) (20.1379, 0.3531) (20.1835, 0.3718) (20.2291, 0.3908) (20.2746, 0.4102) (20.3201, 0.4299) (20.3655, 0.4499) (20.4109, 0.4702) (20.4561, 0.4908) (20.5014, 0.5118) (20.5466, 0.533) (20.5917, 0.5546) (20.6367, 0.5764) (20.6817, 0.5986) (20.7267, 0.6211) (20.7716, 0.6438) (20.8164, 0.6668) (20.8611, 0.6902) (20.9058, 0.7138) (20.9504, 0.7376) (20.995, 0.7618) (21.0395, 0.7863) (21.0839, 0.811) (21.1283, 0.836) (21.1726, 0.8612) (21.2168, 0.8867) (21.261, 0.9125) (21.3051, 0.9386) (21.3491, 0.9649) (21.3931, 0.9915) (21.437, 1.0183) (21.4808, 1.0454) (21.5245, 1.0728) (21.5682, 1.1004) (21.6118, 1.1282) (21.6553, 1.1563) (21.6988, 1.1847) (21.7422, 1.2133) (21.7855, 1.2421) (21.8287, 1.2712) (21.8719, 1.3006) (21.9063, 1.3242) (21.9321, 1.3421) (21.9493, 1.354) (21.9579, 1.36) knots 0 0 0 0 0 0 0.01428571 0.02857143 0.04285714 0.05714286 0.07142857 0.08571429 0.1 0.11428571 0.12857143 0.14285714 0.15714286 0.17142857 0.18571429 0.2 0.21428571 0.22857143 0.24285714 0.25714286 0.27142857 0.28571429 0.3 0.31428571 0.32857143 0.34285714 0.35714286 0.37142857 0.38571429 0.4 0.41428571 0.42857143 0.44285714 0.45714286 0.47142857 0.48571429 0.5 0.51428571 0.52857143 0.54285714 0.55714286 0.57142857 0.58571429 0.6 0.61428571 0.62857143 0.64285714 0.65714286 0.67142857 0.68571429 0.7 0.71428571 0.72857143 0.74285714 0.75714286 0.77142857 0.78571429 0.8 0.81428571 0.82857143 0.84285714 0.85714286 0.87142857 0.88571429 0.9 0.91428571 0.92857143 0.94285714 0.95714286 0.97142857 0.98571429 1 1 1 1 1 1
  line L57 (21.9579, 1.36) -> (21.9041, 2.0524)
  line L58 (21.9041, 2.0524) -> (21.8284, 2.7428)
  spline S29 degree 5 poles (21.8284, 2.7428) (21.8188, 2.747) (21.7997, 2.7556) (21.771, 2.7683) (21.7327, 2.7852) (21.6849, 2.806) (21.637, 2.8265) (21.5891, 2.8468) (21.5412, 2.8669) (21.4932, 2.8867) (21.4452, 2.9062) (21.3972, 2.9255) (21.3491, 2.9445) (21.3011, 2.9632) (21.253, 2.9817) (21.2049, 2.9999) (21.1568, 3.0179) (21.1086, 3.0356) (21.0604, 3.053) (21.0123, 3.0701) (20.964, 3.087) (20.9158, 3.1036) (20.8676, 3.1199) (20.8193, 3.1359) (20.7711, 3.1517) (20.7228, 3.1672) (20.6745, 3.1823) (20.6262, 3.1972) (20.5779, 3.2118) (20.5296, 3.2261) (20.4813, 3.2401) (20.4329, 3.2539) (20.3846, 3.2673) (20.3363, 3.2804) (20.2879, 3.2932) (20.2396, 3.3057) (20.1913, 3.3179) (20.1429, 3.3297) (20.0946, 3.3413) (20.0462, 3.3525) (19.9979, 3.3634) (19.9496, 3.3739) (19.9013, 3.3842) (19.853, 3.3941) (19.8047, 3.4036) (19.7564, 3.4128) (19.7081, 3.4216) (19.6599, 3.4301) (19.6116, 3.4382) (19.5634, 3.446) (19.5152, 3.4533) (19.467, 3.4603) (19.4189, 3.4669) (19.3707, 3.4731) (19.3226, 3.4789) (19.2746, 3.4843) (19.2265, 3.4892) (19.1786, 3.4937) (19.1306, 3.4977) (19.0827, 3.5012) (19.0349, 3.5043) (18.987, 3.5069) (18.9393, 3.509) (18.8916, 3.5106) (18.8439, 3.5117) (18.7963, 3.5121) (18.7489, 3.5118) (18.7015, 3.5107) (18.6543, 3.5087) (18.6072, 3.5058) (18.5602, 3.502) (18.5227, 3.4982) (18.4947, 3.4949) (18.476, 3.4926) (18.4667, 3.4913) knots -1 -1 -1 -1 -1 -1 -0.98571429 -0.97142857 -0.95714286 -0.94285714 -0.92857143 -0.91428571 -0.9 -0.88571429 -0.87142857 -0.85714286 -0.84285714 -0.82857143 -0.81428571 -0.8 -0.78571429 -0.77142857 -0.75714286 -0.74285714 -0.72857143 -0.71428571 -0.7 -0.68571429 -0.67142857 -0.65714286 -0.64285714 -0.62857143 -0.61428571 -0.6 -0.58571429 -0.57142857 -0.55714286 -0.54285714 -0.52857143 -0.51428571 -0.5 -0.48571429 -0.47142857 -0.45714286 -0.44285714 -0.42857143 -0.41428571 -0.4 -0.38571429 -0.37142857 -0.35714286 -0.34285714 -0.32857143 -0.31428571 -0.3 -0.28571429 -0.27142857 -0.25714286 -0.24285714 -0.22857143 -0.21428571 -0.2 -0.18571429 -0.17142857 -0.15714286 -0.14285714 -0.12857143 -0.11428571 -0.1 -0.08571429 -0.07142857 -0.05714286 -0.04285714 -0.02857143 -0.01428571 0 0 0 0 0 0
  line L59 (18.4667, 3.4913) -> (17.6799, 3.3426)
  arc A44 (17.0984, 3.7274) -> (17.6799, 3.3426) centre (17.587, 3.8339) ccw
  arc A45 (17.0984, 3.7274) -> (16.7873, 4.9434) centre (0, 0) ccw
  arc A46 (17.1124, 5.5602) -> (16.7873, 4.9434) centre (17.2669, 5.0846) ccw
  line L60 (17.1124, 5.5602) -> (17.874, 5.8076)
  spline S30 degree 5 poles (17.874, 5.8076) (17.8828, 5.811) (17.9003, 5.8179) (17.9265, 5.8285) (17.9612, 5.8431) (18.0042, 5.8623) (18.0469, 5.8825) (18.0893, 5.9034) (18.1313, 5.9252) (18.1731, 5.9477) (18.2146, 5.9709) (18.2559, 5.9947) (18.297, 6.0191) (18.3379, 6.0439) (18.3786, 6.0691) (18.4191, 6.0948) (18.4594, 6.1209) (18.4995, 6.1475) (18.5395, 6.1744) (18.5792, 6.2018) (18.6188, 6.2296) (18.6582, 6.2578) (18.6974, 6.2864) (18.7365, 6.3153) (18.7754, 6.3445) (18.8141, 6.3742) (18.8527, 6.4041) (18.8911, 6.4344) (18.9294, 6.465) (18.9675, 6.4959) (19.0054, 6.5272) (19.0432, 6.5588) (19.0808, 6.5907) (19.1183, 6.6228) (19.1556, 6.6553) (19.1927, 6.6881) (19.2297, 6.7211) (19.2666, 6.7545) (19.3033, 6.7881) (19.3398, 6.822) (19.3762, 6.8562) (19.4125, 6.8906) (19.4486, 6.9253) (19.4845, 6.9603) (19.5203, 6.9956) (19.556, 7.0311) (19.5915, 7.0668) (19.6268, 7.1028) (19.6621, 7.1391) (19.6971, 7.1756) (19.732, 7.2123) (19.7668, 7.2493) (19.8014, 7.2866) (19.8359, 7.324) (19.8702, 7.3618) (19.9044, 7.3997) (19.9384, 7.4379) (19.9723, 7.4763) (20.006, 7.5149) (20.0396, 7.5538) (20.0731, 7.5929) (20.1064, 7.6322) (20.1395, 7.6717) (20.1725, 7.7115) (20.2054, 7.7514) (20.2381, 7.7916) (20.2707, 7.832) (20.3031, 7.8726) (20.3354, 7.9134) (20.3675, 7.9545) (20.3995, 7.9957) (20.4249, 8.0288) (20.444, 8.0538) (20.4566, 8.0705) (20.463, 8.0788) knots 0 0 0 0 0 0 0.01428571 0.02857143 0.04285714 0.05714286 0.07142857 0.08571429 0.1 0.11428571 0.12857143 0.14285714 0.15714286 0.17142857 0.18571429 0.2 0.21428571 0.22857143 0.24285714 0.25714286 0.27142857 0.28571429 0.3 0.31428571 0.32857143 0.34285714 0.35714286 0.37142857 0.38571429 0.4 0.41428571 0.42857143 0.44285714 0.45714286 0.47142857 0.48571429 0.5 0.51428571 0.52857143 0.54285714 0.55714286 0.57142857 0.58571429 0.6 0.61428571 0.62857143 0.64285714 0.65714286 0.67142857 0.68571429 0.7 0.71428571 0.72857143 0.74285714 0.75714286 0.77142857 0.78571429 0.8 0.81428571 0.82857143 0.84285714 0.85714286 0.87142857 0.88571429 0.9 0.91428571 0.92857143 0.94285714 0.95714286 0.97142857 0.98571429 1 1 1 1 1 1
  line L61 (20.463, 8.0788) -> (20.1978, 8.7207)
  line L62 (20.1978, 8.7207) -> (19.9124, 9.3539)
  spline S31 degree 5 poles (19.9124, 9.3539) (19.902, 9.355) (19.8812, 9.3572) (19.85, 9.3605) (19.8084, 9.3647) (19.7565, 9.3697) (19.7046, 9.3744) (19.6527, 9.3789) (19.6009, 9.3832) (19.5492, 9.3872) (19.4975, 9.3909) (19.4459, 9.3944) (19.3943, 9.3976) (19.3428, 9.4006) (19.2914, 9.4033) (19.24, 9.4058) (19.1887, 9.408) (19.1374, 9.4099) (19.0862, 9.4116) (19.0351, 9.413) (18.9841, 9.4142) (18.9331, 9.415) (18.8822, 9.4156) (18.8313, 9.416) (18.7805, 9.416) (18.7299, 9.4158) (18.6792, 9.4154) (18.6287, 9.4146) (18.5783, 9.4136) (18.5279, 9.4122) (18.4776, 9.4106) (18.4274, 9.4087) (18.3773, 9.4065) (18.3273, 9.4041) (18.2773, 9.4013) (18.2275, 9.3983) (18.1778, 9.3949) (18.1281, 9.3913) (18.0786, 9.3873) (18.0291, 9.383) (17.9798, 9.3784) (17.9306, 9.3736) (17.8815, 9.3684) (17.8325, 9.3628) (17.7836, 9.357) (17.7348, 9.3508) (17.6862, 9.3443) (17.6377, 9.3375) (17.5893, 9.3303) (17.541, 9.3227) (17.4929, 9.3148) (17.4449, 9.3066) (17.3971, 9.298) (17.3494, 9.289) (17.3019, 9.2797) (17.2545, 9.2699) (17.2073, 9.2598) (17.1603, 9.2492) (17.1134, 9.2382) (17.0668, 9.2267) (17.0203, 9.2149) (16.9741, 9.2026) (16.928, 9.1898) (16.8821, 9.1766) (16.8365, 9.1629) (16.7911, 9.1486) (16.746, 9.1336) (16.7013, 9.1179) (16.657, 9.1015) (16.6131, 9.0842) (16.5696, 9.066) (16.5352, 9.0508) (16.5095, 9.0391) (16.4925, 9.031) (16.484, 9.027) knots -1 -1 -1 -1 -1 -1 -0.98571429 -0.97142857 -0.95714286 -0.94285714 -0.92857143 -0.91428571 -0.9 -0.88571429 -0.87142857 -0.85714286 -0.84285714 -0.82857143 -0.81428571 -0.8 -0.78571429 -0.77142857 -0.75714286 -0.74285714 -0.72857143 -0.71428571 -0.7 -0.68571429 -0.67142857 -0.65714286 -0.64285714 -0.62857143 -0.61428571 -0.6 -0.58571429 -0.57142857 -0.55714286 -0.54285714 -0.52857143 -0.51428571 -0.5 -0.48571429 -0.47142857 -0.45714286 -0.44285714 -0.42857143 -0.41428571 -0.4 -0.38571429 -0.37142857 -0.35714286 -0.34285714 -0.32857143 -0.31428571 -0.3 -0.28571429 -0.27142857 -0.25714286 -0.24285714 -0.22857143 -0.21428571 -0.2 -0.18571429 -0.17142857 -0.15714286 -0.14285714 -0.12857143 -0.11428571 -0.1 -0.08571429 -0.07142857 -0.05714286 -0.04285714 -0.02857143 -0.01428571 0 0 0 0 0 0
  line L63 (16.484, 9.027) -> (15.7816, 8.6423)
  arc A47 (15.1098, 8.8286) -> (15.7816, 8.6423) centre (15.5415, 9.0809) ccw
  arc A48 (15.1098, 8.8286) -> (14.4381, 9.889) centre (0, 0) ccw
  arc A49 (14.5567, 10.5761) -> (14.4381, 9.889) centre (14.8506, 10.1715) ccw
  line L64 (14.5567, 10.5761) -> (15.2045, 11.0467)
  spline S32 degree 5 poles (15.2045, 11.0467) (15.2118, 11.0527) (15.2264, 11.0646) (15.248, 11.0828) (15.2764, 11.1074) (15.3114, 11.139) (15.3458, 11.1713) (15.3796, 11.2044) (15.4129, 11.2381) (15.4457, 11.2724) (15.478, 11.3073) (15.5099, 11.3427) (15.5415, 11.3786) (15.5727, 11.4148) (15.6036, 11.4514) (15.6342, 11.4883) (15.6644, 11.5256) (15.6944, 11.5632) (15.7241, 11.6012) (15.7534, 11.6396) (15.7825, 11.6782) (15.8112, 11.7172) (15.8397, 11.7565) (15.8679, 11.7961) (15.8959, 11.8359) (15.9236, 11.8761) (15.951, 11.9165) (15.9782, 11.9571) (16.0051, 11.9981) (16.0318, 12.0393) (16.0582, 12.0807) (16.0844, 12.1224) (16.1103, 12.1644) (16.136, 12.2066) (16.1614, 12.249) (16.1866, 12.2916) (16.2116, 12.3345) (16.2364, 12.3776) (16.2609, 12.4209) (16.2852, 12.4644) (16.3092, 12.5082) (16.333, 12.5522) (16.3567, 12.5963) (16.38, 12.6407) (16.4032, 12.6853) (16.4261, 12.7301) (16.4489, 12.775) (16.4713, 12.8202) (16.4936, 12.8656) (16.5157, 12.9111) (16.5375, 12.9569) (16.5592, 13.0028) (16.5806, 13.0489) (16.6018, 13.0952) (16.6228, 13.1417) (16.6436, 13.1883) (16.6641, 13.2352) (16.6845, 13.2822) (16.7046, 13.3293) (16.7246, 13.3767) (16.7443, 13.4242) (16.7638, 13.4719) (16.7831, 13.5197) (16.8023, 13.5677) (16.8212, 13.6159) (16.8398, 13.6642) (16.8583, 13.7127) (16.8766, 13.7613) (16.8947, 13.8101) (16.9126, 13.859) (16.9302, 13.9081) (16.9442, 13.9475) (16.9546, 13.9772) (16.9615, 13.9969) (16.9649, 14.0068) knots 0 0 0 0 0 0 0.01428571 0.02857143 0.04285714 0.05714286 0.07142857 0.08571429 0.1 0.11428571 0.12857143 0.14285714 0.15714286 0.17142857 0.18571429 0.2 0.21428571 0.22857143 0.24285714 0.25714286 0.27142857 0.28571429 0.3 0.31428571 0.32857143 0.34285714 0.35714286 0.37142857 0.38571429 0.4 0.41428571 0.42857143 0.44285714 0.45714286 0.47142857 0.48571429 0.5 0.51428571 0.52857143 0.54285714 0.55714286 0.57142857 0.58571429 0.6 0.61428571 0.62857143 0.64285714 0.65714286 0.67142857 0.68571429 0.7 0.71428571 0.72857143 0.74285714 0.75714286 0.77142857 0.78571429 0.8 0.81428571 0.82857143 0.84285714 0.85714286 0.87142857 0.88571429 0.9 0.91428571 0.92857143 0.94285714 0.95714286 0.97142857 0.98571429 1 1 1 1 1 1
  line L65 (16.9649, 14.0068) -> (16.5144, 14.5353)
  line L66 (16.5144, 14.5353) -> (16.0474, 15.0493)
  spline S33 degree 5 poles (16.0474, 15.0493) (16.0371, 15.0472) (16.0166, 15.0429) (15.9859, 15.0363) (15.9451, 15.0275) (15.8941, 15.0162) (15.8433, 15.0046) (15.7926, 14.9929) (15.7421, 14.9809) (15.6916, 14.9688) (15.6413, 14.9564) (15.5911, 14.9437) (15.5411, 14.9309) (15.4912, 14.9178) (15.4414, 14.9045) (15.3918, 14.8909) (15.3423, 14.8772) (15.293, 14.8632) (15.2437, 14.8489) (15.1947, 14.8345) (15.1458, 14.8198) (15.097, 14.8049) (15.0484, 14.7897) (14.9999, 14.7743) (14.9516, 14.7587) (14.9035, 14.7428) (14.8555, 14.7267) (14.8077, 14.7104) (14.76, 14.6938) (14.7125, 14.677) (14.6652, 14.6599) (14.618, 14.6426) (14.571, 14.6251) (14.5242, 14.6072) (14.4776, 14.5892) (14.4312, 14.5709) (14.3849, 14.5523) (14.3388, 14.5335) (14.2929, 14.5144) (14.2472, 14.4951) (14.2017, 14.4755) (14.1564, 14.4556) (14.1113, 14.4355) (14.0664, 14.4151) (14.0217, 14.3945) (13.9773, 14.3735) (13.933, 14.3523) (13.889, 14.3308) (13.8452, 14.309) (13.8016, 14.2869) (13.7583, 14.2645) (13.7152, 14.2419) (13.6724, 14.2189) (13.6298, 14.1956) (13.5875, 14.1721) (13.5454, 14.1482) (13.5037, 14.1239) (13.4622, 14.0993) (13.4211, 14.0744) (13.3803, 14.0491) (13.3397, 14.0234) (13.2995, 13.9974) (13.2596, 13.9711) (13.2201, 13.9443) (13.1809, 13.9172) (13.1422, 13.8896) (13.104, 13.8614) (13.0663, 13.8327) (13.0293, 13.8033) (12.9928, 13.7733) (12.9571, 13.7426) (12.929, 13.7175) (12.9083, 13.6984) (12.8946, 13.6855) (12.8877, 13.679) knots -1 -1 -1 -1 -1 -1 -0.98571429 -0.97142857 -0.95714286 -0.94285714 -0.92857143 -0.91428571 -0.9 -0.88571429 -0.87142857 -0.85714286 -0.84285714 -0.82857143 -0.81428571 -0.8 -0.78571429 -0.77142857 -0.75714286 -0.74285714 -0.72857143 -0.71428571 -0.7 -0.68571429 -0.67142857 -0.65714286 -0.64285714 -0.62857143 -0.61428571 -0.6 -0.58571429 -0.57142857 -0.55714286 -0.54285714 -0.52857143 -0.51428571 -0.5 -0.48571429 -0.47142857 -0.45714286 -0.44285714 -0.42857143 -0.41428571 -0.4 -0.38571429 -0.37142857 -0.35714286 -0.34285714 -0.32857143 -0.31428571 -0.3 -0.28571429 -0.27142857 -0.25714286 -0.24285714 -0.22857143 -0.21428571 -0.2 -0.18571429 -0.17142857 -0.15714286 -0.14285714 -0.12857143 -0.11428571 -0.1 -0.08571429 -0.07142857 -0.05714286 -0.04285714 -0.02857143 -0.01428571 0 0 0 0 0 0
  line L67 (12.8877, 13.679) -> (12.3386, 13.0961)
  arc A50 (11.642, 13.0657) -> (12.3386, 13.0961) centre (11.9747, 13.439) ccw
  arc A51 (11.642, 13.0657) -> (10.6755, 13.8666) centre (0, 0) ccw
  arc A52 (10.5761, 14.5567) -> (10.6755, 13.8666) centre (10.9806, 14.2628) ccw
  line L68 (10.5761, 14.5567) -> (11.0467, 15.2045)
  spline S34 degree 5 poles (11.0467, 15.2045) (11.0519, 15.2124) (11.062, 15.2283) (11.0769, 15.2522) (11.0964, 15.2845) (11.1199, 15.3253) (11.1426, 15.3667) (11.1646, 15.4086) (11.1858, 15.4509) (11.2064, 15.4937) (11.2263, 15.5369) (11.2457, 15.5804) (11.2647, 15.6242) (11.2831, 15.6683) (11.3012, 15.7127) (11.3189, 15.7573) (11.3362, 15.8021) (11.353, 15.8471) (11.3695, 15.8924) (11.3856, 15.938) (11.4012, 15.9837) (11.4165, 16.0297) (11.4315, 16.0758) (11.4461, 16.1222) (11.4604, 16.1687) (11.4743, 16.2155) (11.4879, 16.2624) (11.5012, 16.3094) (11.5141, 16.3567) (11.5268, 16.4041) (11.5391, 16.4517) (11.5511, 16.4995) (11.5628, 16.5474) (11.5742, 16.5954) (11.5853, 16.6436) (11.5961, 16.692) (11.6066, 16.7405) (11.6168, 16.7891) (11.6267, 16.8379) (11.6364, 16.8868) (11.6457, 16.9358) (11.6548, 16.985) (11.6636, 17.0343) (11.6721, 17.0837) (11.6804, 17.1333) (11.6884, 17.183) (11.6961, 17.2328) (11.7035, 17.2827) (11.7107, 17.3327) (11.7176, 17.3828) (11.7242, 17.4331) (11.7306, 17.4835) (11.7367, 17.5339) (11.7426, 17.5845) (11.7482, 17.6352) (11.7536, 17.686) (11.7586, 17.7369) (11.7635, 17.7879) (11.7681, 17.839) (11.7724, 17.8902) (11.7765, 17.9414) (11.7803, 17.9928) (11.7839, 18.0443) (11.7872, 18.0958) (11.7903, 18.1475) (11.7932, 18.1992) (11.7958, 18.251) (11.7981, 18.3029) (11.8003, 18.3549) (11.8021, 18.407) (11.8038, 18.4592) (11.8049, 18.5009) (11.8056, 18.5323) (11.8061, 18.5533) (11.8063, 18.5637) knots 0 0 0 0 0 0 0.01428571 0.02857143 0.04285714 0.05714286 0.07142857 0.08571429 0.1 0.11428571 0.12857143 0.14285714 0.15714286 0.17142857 0.18571429 0.2 0.21428571 0.22857143 0.24285714 0.25714286 0.27142857 0.28571429 0.3 0.31428571 0.32857143 0.34285714 0.35714286 0.37142857 0.38571429 0.4 0.41428571 0.42857143 0.44285714 0.45714286 0.47142857 0.48571429 0.5 0.51428571 0.52857143 0.54285714 0.55714286 0.57142857 0.58571429 0.6 0.61428571 0.62857143 0.64285714 0.65714286 0.67142857 0.68571429 0.7 0.71428571 0.72857143 0.74285714 0.75714286 0.77142857 0.78571429 0.8 0.81428571 0.82857143 0.84285714 0.85714286 0.87142857 0.88571429 0.9 0.91428571 0.92857143 0.94285714 0.95714286 0.97142857 0.98571429 1 1 1 1 1 1
  line L69 (11.8063, 18.5637) -> (11.2144, 18.9271)
  line L70 (11.2144, 18.9271) -> (10.6114, 19.2717)